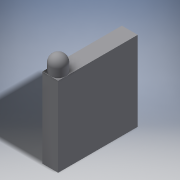
# Autodesk Inventor part: rotation 2
Saved by Autodesk Inventor 2019 (Build 230136000, 136)
## iProperties
Created: 2020-03-28
Part Number: rotation 2
Material: Generic
Document SubType Name: Modeling
Designer: Pulag
Density: 1 g/cm^3
Appearance: Default
Author: Pulag
Autodesk Inventor part; units mm, degrees
ref_plane "YZ Plane" through (0, 0, 0) normal (1, 0, 0) x (0, 1, 0)
ref_plane "XZ Plane" through (0, 0, 0) normal (0, 1, 0) x (-1, 0, 0)
ref_plane "XY Plane" through (0, 0, 0) normal (0, 0, 1) x (1, 0, 0)
sketch "Sketch4" plane through (0, 0, 0) normal (0, 1, 0) x (-1, 0, 0)
  line L0 (0.2787, -1.1584) -> (-1.2213, -1.1584)
  line L1 (-0.149, -2.4672) -> (-1.649, -2.4672)
  line L2 (0.2787, -1.1584) -> (-0.149, -2.4672)
  line L3 (-1.2213, -1.1584) -> (-1.649, -2.4672)
  point P0 (0, 0)
  dimension "d11" = 1.5
  constraints: 8 end point, 2 parallel, 1 horizontal
  measures "d11" distance of L1.start L1.end
extrude "Extrusion4" add sketch "Sketch4" along normal blind 3
body "Solid2"
